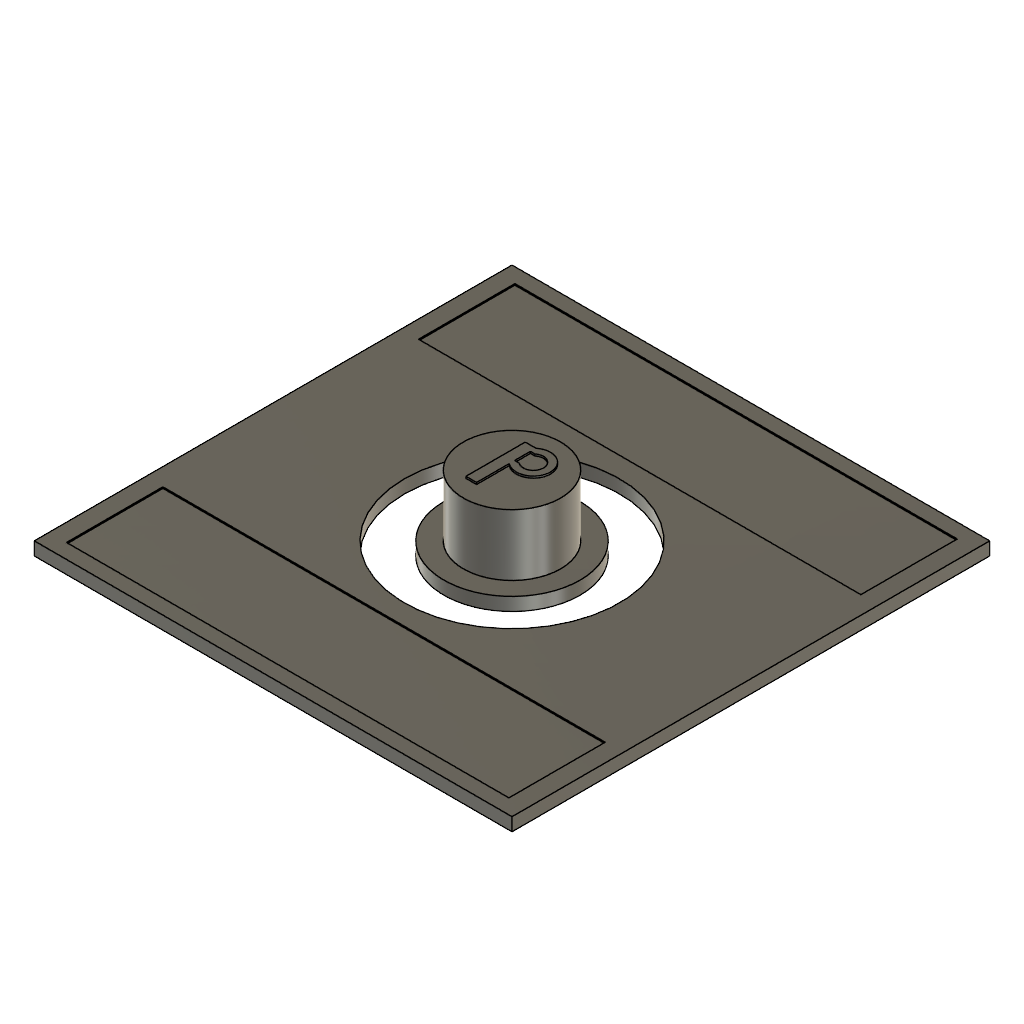
The Real Power Stencil (Autodesk Fusion 360 design; units mm, degrees)
Autodesk Fusion 360 part; units mm, degrees
sketch "Sketch1" plane through (0, 0, 0) normal (0, 0, 1) x (1, 0, 0)
  circle A0 centre (0, 0) radius 7.775
  circle A1 centre (0, 0) radius 12.275
  line L0 (0, 12.275) -> (0, 27.275)
  line L1 (-12.275, 0) -> (-27.275, 0)
  line L2 (-27.275, 0) -> (-27.275, 27.275)
  line L3 (-27.275, 27.275) -> (27.275, 27.275)
  line L4 (27.275, 27.275) -> (27.275, -27.275)
  line L5 (27.275, -27.275) -> (-27.275, -27.275)
  line L6 (-27.275, -27.275) -> (-27.275, 27.275)
  dimension "d1" = 15.55
  dimension "d2" = 4.5
  dimension "d3" = 15
  dimension "d4" = 15
  dimension "d5" = 54.55
  dimension "d6" = 54.55
  constraint coincident A0.centre A1.centre
  constraint coincident A1 L0.start
  constraint vertical L0
  constraint coincident A1 L1.start
  constraint horizontal L1
  constraint perpendicular L1 L2
  constraint horizontal L3
  constraint vertical L4
  constraint horizontal L5
  constraint vertical L6
  measures "d1" diameter of A0
  measures "d3" distance of L0.start L0.end
  measures "d4" distance of L1.start L1.end
  measures "d5" distance of L2.end L3.end
  measures "d6" distance of L2.end L5.end
extrude "Extrude1" add sketch "Sketch1" along normal blind 1.5 contours A0 | A1 L0 L1 L3 L4 L5 L6 | A1 L0 L1 L2 L3 L6 makes body 1 at (-0.3058, -22.2636, 0) makes body 2 at (-1.6159, 2.7988, 0)
sketch "Sketch2" plane through (0, 0, 1.5) normal (0, 0, 1) x (-1, 0, 0)
  circle A0 centre (0, 0) radius 7.775
  line L0 (5.0002, -4.6813) -> (-4.9998, -4.6813)
  line L1 (-4.9998, -4.6813) -> (-4.9998, 4.8187)
  line L2 (-4.9998, 4.8187) -> (5.0002, 4.8187)
  line L3 (5.0002, 4.8187) -> (5.0002, -4.6813)
  line L4 (25.2649, -25.5924) -> (-25.2351, -25.5924)
  line L5 (-25.2351, -25.5924) -> (-25.2351, -14.5924)
  line L6 (-25.2351, -14.5924) -> (25.2649, -14.5924)
  line L7 (25.2649, -14.5924) -> (25.2649, -25.5924)
  line L8 (0, 0) -> (-1.8837, 0)
  line L9 (25.2649, 25.5924) -> (-25.2351, 25.5924)
  line L10 (-25.2351, 25.5924) -> (-25.2351, 14.5924)
  line L11 (-25.2351, 14.5924) -> (25.2649, 14.5924)
  line L12 (25.2649, 14.5924) -> (25.2649, 25.5924)
  dimension "d9" = 10
  dimension "d10" = 9.5
  dimension "d11" = 50.5
  dimension "d12" = 11
  constraint horizontal L0
  constraint vertical L1
  constraint horizontal L2
  constraint vertical L3
  constraint horizontal L4
  constraint vertical L5
  constraint horizontal L6
  constraint vertical L7
  constraint coincident A0.centre L8.start
  constraint horizontal L8
  constraint symmetric L4.start L8 L9.start
  constraint symmetric L4.end L8 L9.end
  constraint symmetric L5.end L8 L10.end
  constraint symmetric L6.end L8 L11.end
  measures "d9" distance of L0.start L0.end
  measures "d10" distance of L0.start L2.end
  measures "d11" distance of L4.start L4.end
  measures "d12" distance of L4.start L6.end
extrude "Extrude2" cut sketch "Sketch2" against normal blind 0.15 contours L0 L1 L2 L3 | L4 L5 L6 L7 | L9 L10 L11 L12 bodies 1 2
extrude "Extrude3" add 1 faces at (-1.6669, 1.5146, 1.35) along direction (0, 0, 1) blind 0.15 on bodies 2 bodies 2
sketch "Sketch3" plane through (0, 0, 1.5) normal (0, 0, 1) x (-1, 0, 0)
  circle A0 centre (0, 0) radius 7.775
  circle A1 centre (0, 0) radius 5.55
  dimension "d17" = 11.1
  constraint coincident A0.centre A1.centre
  measures "d17" diameter of A1
extrude "Extrude4" add sketch "Sketch3" along normal blind 7 contours A1 bodies 2
sketch "Sketch4" plane through (0, 0, 8.5) normal (0, 0, 1) x (-1, 0, 0)
  circle A0 centre (0, 0) radius 5.55
  line L0 (1.8078, -3.3179) -> (1.8078, 3.4555)
  line L1 (1.8078, 3.4555) -> (0.5916, 3.4555)
  line L2 (0.5916, 3.4555) -> (0.5916, -0.2775)
  line L3 (1.8078, -3.3179) -> (0.5916, -3.3179)
  line L4 (0.5916, -0.2775) -> (0.5916, -3.3179)
  arc A1 (0.5916, -0.2775) -> (0.5916, -3.3179) centre (-0.6427, -1.7977) ccw
  arc A2 (0.0874, -0.8986) -> (0.0874, -2.6969) centre (-0.6427, -1.7977) ccw
  line L5 (0.0874, -0.8986) -> (0.5916, -0.8986)
  line L6 (0.0874, -2.6969) -> (0.5916, -2.6969)
  dimension "d20" = -0.8
  constraint vertical L0
  constraint perpendicular L0 L1
  constraint perpendicular L1 L2
  constraint perpendicular L2 L3
  constraint perpendicular L3 L4
  constraint coincident L4 L5.end
  constraint perpendicular L4 L5
  constraint coincident L4 L6.end
  constraint perpendicular L4 L6
extrude "Extrude5" add sketch "Sketch4" along normal blind 0.2 contours L0 L1 L2 L3 L4 | L4 A1 A2 L5 L6 bodies 2
equation "d1 = 11.05 mm + 4.5 mm"
